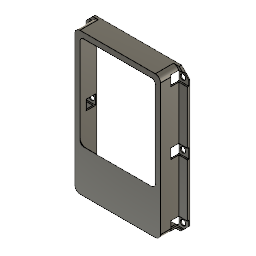
2004699B-exact (Autodesk Fusion 360 design; units mm, degrees)
Autodesk Fusion 360 part; units mm, degrees
sketch "Front" plane through (0, 0, 0) normal (0, 1, 0) x (1, 0, 0) in component "2004699B"
  line L0 (-34.4613, 0.7342) -> (100.7673, 0.7342) construction
  line L1 (-34.854, -115.3184) -> (120.0108, -115.3184) construction
  line L2 (39.1093, -14.9122) -> (120.6654, -14.9122) construction
  line L3 (3.575, 24.5274) -> (3.575, -141.9882) construction
  line L4 (78.251, 23.8729) -> (78.251, -119.9956) construction
  line L5 (-16.7886, -108.2138) -> (88.0691, -108.2138) construction
  line L6 (-18.2286, -5.0898) -> (85.3201, -5.0898) construction
  line L7 (-8.6723, -56.6518) -> (96.0546, -56.6518) construction
  line L8 (-24.3813, -113.9722) -> (90.4255, -113.9722) construction
  line L9 (-27.0881, -0.4088) -> (83.5136, -0.4088) construction
  line L10 (10.2552, -130.527) -> (10.2552, 10.1996) construction
  line L11 (71.52, -130.1852) -> (71.52, 12.6775) construction
  line L12 (5.7848, -130.0998) -> (5.7848, 6.3546) construction
  line L13 (83.0008, -137.1267) -> (83.0008, 10.6162) construction
  line L14 (-1.2002, -137.339) -> (-1.2002, 17.644) construction
  line L15 (110.5413, -110.6956) -> (5.7848, -110.6956) construction
  line L16 (110.1974, -34.3178) -> (-2.9547, -34.3178) construction
  line L17 (102.8889, -60.7158) -> (-8.8875, -60.7158) construction
  line L18 (102.459, -52.5878) -> (-11.4669, -52.5878) construction
  line L19 (40.913, -17.1802) -> (40.913, 17.1835) construction
  line L20 (69.6478, 8.6501) -> (89.4046, -11.1067) construction
  line L21 (-5.4342, -8.9542) -> (10.2552, 6.7154) construction
  line L22 (-6.1303, -103.6453) -> (12.6902, -122.4658) construction
  line L23 (73.7302, -117.8806) -> (90.3753, -101.2137) construction
  line L24 (-2.868, -104.1498) -> (87.443, -104.1498) construction
  line L25 (-3.4391, -112.2778) -> (87.0011, -112.2778) construction
  line L26 (-3.1536, -9.1538) -> (86.0732, -9.1538) construction
  line L27 (-3.3677, -1.0258) -> (85.288, -1.0258) construction
  line L28 (10.2552, -110.6956) -> (71.52, -110.6956)
  line L29 (71.52, -110.6956) -> (71.52, -34.3178)
  line L30 (71.52, -34.3178) -> (10.2552, -34.3178)
  line L31 (10.2552, -34.3178) -> (10.2552, -110.6956)
  line L32 (-1.2002, -115.3184) -> (83.0008, -115.3184)
  line L33 (83.0008, -115.3184) -> (83.0008, 0.7342)
  line L34 (83.0008, 0.7342) -> (-1.2002, 0.7342)
  line L35 (-1.2002, 0.7342) -> (-1.2002, -115.3184)
  line L36 (76.0158, -119.9569) -> (76.0158, 9.6762) construction
  line L37 (5.7848, -115.3184) -> (76.0222, -115.3184) construction
  line L38 (76.0222, -115.3184) -> (76.0222, 0.7342) construction
  line L39 (76.0222, 0.7342) -> (5.7848, 0.7342) construction
  line L40 (5.7848, 0.7342) -> (5.7848, -115.3184) construction
  line L41 (76.0222, 0.7342) -> (5.7848, 0.7342)
  line L42 (5.7848, 0.7342) -> (5.7848, -115.3184)
  line L43 (5.7848, -115.3184) -> (76.0222, -115.3184)
  line L44 (76.0222, -115.3184) -> (76.0222, 0.7342)
  line L45 (-1.2002, -108.5588) -> (5.5429, -115.3184)
  line L46 (76.2891, -115.3184) -> (83.0008, -108.585)
  line L47 (77.5637, 0.7342) -> (83.0008, -4.7029)
  line L48 (4.2664, 0.7342) -> (-1.2002, -4.7255)
  point P0 (3.575, -108.2138)
  point P1 (78.251, -108.2138)
  point P2 (78.251, -56.6518)
  point P3 (78.251, -5.0898)
  point P4 (3.575, -5.0898)
  point P5 (3.575, -56.6518)
  dimension "d1" = 1.143
  dimension "d2" = 116.0526
  dimension "d3" = 113.5634
  dimension "d4" = 103.124
  dimension "d5" = 51.562
  dimension "d6" = 74.676
  dimension "d7" = 2.2098
  dimension "d8" = 4.4704
  dimension "d9" = 61.2648
  dimension "d10" = 84.201
  dimension "d11" = 6.985
  dimension "d12" = 76.3778
  dimension "d13" = 4.6228
  dimension "d14" = 100.4062
  dimension "d15" = 37.338
  dimension "d16" = 8.128
  dimension "d17" = 4.064
  dimension "d18" = 3.6322
  dimension "d19" = 3.6322
  dimension "d20" = 3.6322
  dimension "d21" = 3.6322
  dimension "d22" = 4.064
  dimension "d23" = 8.128
  dimension "d25" = 4.064
  dimension "d26" = 8.128
  dimension "d27" = 70.231
  constraint horizontal L0
  constraint horizontal L1
  constraint horizontal L2
  constraint perpendicular L1 L3
  constraint perpendicular L1 L4
  constraint perpendicular L4 L5
  constraint perpendicular L4 L6
  constraint perpendicular L4 L7
  constraint parallel L1 L8
  constraint perpendicular L4 L9
  constraint perpendicular L0 L10
  constraint perpendicular L1 L11
  constraint perpendicular L0 L12
  constraint perpendicular L5 L13
  constraint perpendicular L6 L14
  constraint coincident L12 L15.end
  constraint perpendicular L12 L15
  constraint perpendicular L14 L16
  constraint perpendicular L14 L17
  constraint perpendicular L14 L18
  constraint perpendicular L9 L19
  constraint coincident L10 L21.end
  constraint coincident L5 P0
  constraint coincident L3 P0
  constraint coincident L4 P1
  constraint coincident L5 P1
  constraint coincident L7 P2
  constraint coincident L4 P2
  constraint coincident L6 P3
  constraint coincident L4 P3
  constraint coincident L6 P4
  constraint coincident L3 P4
  constraint coincident L7 P5
  constraint coincident L3 P5
  constraint coincident L23 L24.end
  constraint perpendicular L13 L24
  constraint perpendicular L13 L25
  constraint perpendicular L13 L26
  constraint perpendicular L13 L27
  constraint horizontal L28
  constraint vertical L29
  constraint horizontal L30
  constraint vertical L31
  constraint coincident L16 L29.end
  constraint coincident L11 L29.end
  constraint coincident L10 L28.start
  constraint coincident L15 L28.start
  constraint horizontal L32
  constraint vertical L33
  constraint horizontal L34
  constraint vertical L35
  constraint coincident L0 L33.end
  constraint coincident L13 L33.end
  constraint coincident L1 L32.start
  constraint coincident L14 L32.start
  constraint perpendicular L0 L36
  constraint horizontal L37
  constraint vertical L38
  constraint horizontal L39
  constraint vertical L40
  constraint coincident L0 L38.end
  constraint coincident L12 L37.start
  constraint coincident L32 L37.start
  constraint horizontal L41
  constraint vertical L42
  constraint horizontal L43
  constraint vertical L44
  constraint coincident L14 L45.start
  constraint coincident L1 L45.end
  constraint coincident L22 L45.end
  constraint coincident L23 L46.start
  constraint coincident L32 L46.start
  constraint coincident L13 L46.end
  constraint coincident L20 L47.start
  constraint coincident L34 L47.start
  constraint coincident L13 L47.end
  constraint coincident L20 L47.end
  constraint coincident L34 L48.start
  constraint coincident L21 L48.start
  constraint coincident L21 L48.end
  constraint coincident L35 L48.end
  measures "d1" distance of L0 L9
  measures "d2" distance of L0 L1
  measures "d3" distance of L8 L9
  measures "d4" distance of L5 L6
  measures "d5" distance of L6 L7
  measures "d6" distance of L3 L4
  measures "d7" distance of L3 L12
  measures "d8" distance of L10 L12
  measures "d9" distance of L10 L11
  measures "d10" distance of L13 L14
  measures "d11" distance of L12 L14
  measures "d12" distance of L15 L16
  measures "d13" distance of L1 L15
  measures "d14" distance of L1 L2
  measures "d15" distance of L3 L19
  measures "d16" distance of L17 L18
  measures "d17" distance of L7 L18
  measures "d18" distance of L20 P3
  measures "d19" distance of L21 P4
  measures "d20" distance of L22 P0
  measures "d21" distance of L23 P1
  measures "d22" distance of L5 L25
  measures "d23" distance of L24 L25
  measures "d25" distance of L6 L27
  measures "d26" distance of L26 L27
  measures "d27" distance of L12 L36
extrude "Extrude1" add sketch "Front" against normal blind 17.0434 contours L32 L34 L41 L42 L43 L44 in component "2004699B"
extrude "Extrude2" add sketch "Front" against normal blind 2.0828 contours L32 L34 L35 L42 L45 L48 | L32 L33 L34 L44 L46 L47 in component "2004699B"
fillet "Fillet1" radius 4.318 4 edges at (5.7848, -9.5631, -0.7342) (76.0222, -9.5631, -0.7342) (76.0222, -9.5631, 115.3184) (5.7848, -9.5631, 115.3184) in component "2004699B"
fillet "Fillet2" radius 2.8194 4 edges at (71.52, -8.5217, 110.6956) (10.2552, -8.5217, 110.6956) (71.52, -8.5217, 34.3178) (10.2552, -8.5217, 34.3178) in component "2004699B"
hole "Hole1" at (78.251, 0, 108.2138) at (78.251, 0, 56.6518) at (78.251, 0, 5.0898) at (3.575, 0, 5.0898) at (3.575, 0, 56.6518) at (3.575, 0, 108.2138) direction (0, -1, 0) diameter 4.3434 end through all in component "2004699B"
sketch "Sketch3" plane through (0, 0, 0) normal (0, 1, 0) x (1, 0, 0) in component "2004699B"
  line L0 (88.5571, -114.1754) -> (-29.017, -114.1754) construction
  line L1 (6.9278, -119.135) -> (6.9278, -3.6092) construction
  line L2 (74.8728, -110.975) -> (74.8728, 6.1599) construction
  line L3 (95.5329, -0.4088) -> (-26.782, -0.4088) construction
  line L4 (-34.4613, 0.7342) -> (100.7673, 0.7342) construction
  line L5 (5.7848, -130.0998) -> (5.7848, 6.3546) construction
  line L6 (-34.854, -115.3184) -> (120.0108, -115.3184) construction
  line L7 (76.0158, -119.9569) -> (76.0158, 9.6762) construction
  line L8 (71.6724, -114.1754) -> (10.1282, -114.1754)
  line L9 (6.9278, -110.975) -> (6.9278, -0.4088)
  line L10 (10.1282, -0.4088) -> (71.6724, -0.4088)
  line L11 (74.8728, -3.6092) -> (74.8728, -114.1754)
  arc A0 (74.8728, -3.6092) -> (71.6724, -0.4088) centre (71.6724, -3.6092) ccw
  arc A1 (10.1282, -0.4088) -> (6.9278, -3.6092) centre (10.1282, -3.6092) ccw
  arc A2 (71.6724, -114.1754) -> (74.8728, -110.975) centre (71.6724, -110.975) ccw
  arc A3 (6.9278, -110.975) -> (10.1282, -114.1754) centre (10.1282, -110.975) ccw
  dimension "d37" = 1.143
  dimension "d38" = 1.143
  dimension "d39" = 1.143
  dimension "d40" = 1.143
  dimension "d41" = 3.2004
  dimension "d42" = 3.2004
  dimension "d43" = 3.2004
  dimension "d44" = 3.2004
  constraint horizontal L0
  constraint perpendicular L0 L1
  constraint perpendicular L0 L2
  constraint perpendicular L2 L3
  constraint horizontal L8
  constraint vertical L9
  constraint horizontal L10
  constraint vertical L11
  constraint coincident L1 L9.end
  constraint coincident L3 L9.end
  constraint coincident L2 L11.end
  constraint coincident L0 L11.end
  constraint tangent L11 A0
  constraint tangent L10 A0
  constraint coincident L9.end L10
  constraint tangent L10 A1
  constraint tangent L1 A1
  constraint coincident L11.end L8
  constraint tangent L2 A2
  constraint tangent L8 A2
  constraint tangent L8 A3
  constraint tangent L9 A3
  measures "d37" distance of L3 L4
  measures "d38" distance of L1 L5
  measures "d39" distance of L0 L6
  measures "d40" distance of L2 L7
  measures "d41" radius of A0
  measures "d42" radius of A1
  measures "d43" radius of A2
  measures "d44" radius of A3
extrude "Extrude3" cut sketch "Sketch3" against normal blind 14.986 in component "2004699B"
chamfer "Chamfer1" distance 2.032 angle 45 8 edges at (40.8876, -14.986, 34.3178) (11.081, -14.986, 35.1436) (10.2552, -14.986, 72.5067) (11.081, -14.986, 109.8698) (40.8876, -14.986, 110.6956) (70.6942, -14.986, 109.8698) (71.52, -14.986, 72.5067) (70.6942, -14.986, 35.1436) in component "2004699B"
sketch "Sketch4" plane through (83.0008, 0, 0) normal (1, 0, 0) x (0, 1, 0) in component "2004699B"
  line L0 (0, 4.7029) -> (0, 108.585)
  line L1 (0, 108.585) -> (-2.0828, 108.585)
  line L2 (-2.0828, 108.585) -> (-2.0828, 4.7029)
  line L3 (-2.0828, 4.7029) -> (0, 4.7029)
  line L4 (-0.9906, 121.8672) -> (-0.9906, -5.2486) construction
  line L5 (0, 108.2121) -> (-3.3976, 108.2121) construction
  line L6 (0, 56.644) -> (-3.817, 56.644) construction
  line L7 (0, 0) -> (-1.1062, 0) construction
  line L8 (1.8872, 112.2761) -> (-9.9271, 112.2761) construction
  line L9 (1.8112, 104.1481) -> (-10.4595, 104.1481) construction
  line L10 (1.71, 60.708) -> (-9.8241, 60.708) construction
  line L11 (2.1656, 52.58) -> (0.9254, 52.58) construction
  line L12 (0.9254, 52.58) -> (-9.5412, 52.58) construction
  line L13 (0, 5.0822) -> (-6.1548, 5.0822) construction
  line L14 (2.1892, 9.1462) -> (-10.0058, 9.1462) construction
  line L15 (2.6197, 1.0182) -> (-10.581, 1.0182) construction
  line L16 (-8.6106, 122.6091) -> (-8.6106, -10.4565) construction
  line L17 (-8.6106, 60.708) -> (-0.9906, 60.708)
  line L18 (-0.9906, 60.708) -> (-0.9906, 52.58)
  line L19 (-0.9906, 52.58) -> (-8.6106, 52.58)
  line L20 (-8.6106, 52.58) -> (-8.6106, 60.708)
  line L21 (-8.6106, 9.1462) -> (-0.9906, 9.1462)
  line L22 (-0.9906, 9.1462) -> (-0.9906, 1.0182)
  line L23 (-0.9906, 1.0182) -> (-8.6106, 1.0182)
  line L24 (-8.6106, 1.0182) -> (-8.6106, 9.1462)
  line L25 (-8.6106, 112.2761) -> (-0.9906, 112.2761)
  line L26 (-0.9906, 112.2761) -> (-0.9906, 104.1481)
  line L27 (-0.9906, 104.1481) -> (-8.6106, 104.1481)
  line L28 (-8.6106, 104.1481) -> (-8.6106, 112.2761)
  point P0 (0, 119.9956)
  dimension "d48" = 0.9906
  dimension "d49" = 4.064
  dimension "d50" = 8.128
  dimension "d51" = 4.064
  dimension "d52" = 8.128
  dimension "d54" = 4.064
  dimension "d55" = 8.128
  dimension "d56" = 7.62
  constraint parallel L2 L4
  constraint coincident L0 L5.start
  constraint perpendicular L2 L5
  constraint midpoint L0 L6.start
  constraint perpendicular L0 L6
  constraint coincident L7.start origin
  constraint perpendicular L4 L7
  constraint perpendicular L4 L8
  constraint perpendicular L2 L9
  constraint perpendicular L0 L10
  constraint perpendicular L4 L11
  constraint perpendicular L4 L12
  constraint coincident L0 L13.start
  constraint perpendicular L0 L13
  constraint perpendicular L0 L14
  constraint perpendicular L0 L15
  constraint perpendicular L12 L16
  constraint horizontal L17
  constraint vertical L18
  constraint horizontal L19
  constraint vertical L20
  constraint coincident L4 L18.end
  constraint coincident L12 L18.end
  constraint coincident L16 L17.start
  constraint coincident L10 L17.start
  constraint horizontal L21
  constraint vertical L22
  constraint horizontal L23
  constraint vertical L24
  constraint coincident L4 L22.end
  constraint coincident L15 L22.end
  constraint coincident L16 L21.start
  constraint coincident L14 L21.start
  constraint horizontal L25
  constraint vertical L26
  constraint horizontal L27
  constraint vertical L28
  constraint coincident L4 L26.end
  constraint coincident L9 L26.end
  constraint coincident L16 L25.start
  constraint coincident L8 L25.start
  measures "d48" distance of L4 P0
  measures "d49" distance of L13 L14
  measures "d50" distance of L14 L15
  measures "d51" distance of L6 L10
  measures "d52" distance of L10 L12
  measures "d54" distance of L5 L9
  measures "d55" distance of L8 L9
  measures "d56" distance of L4 L16
extrude "Extrude4" cut sketch "Sketch4" against normal through all contours L2 L3 L21 L22 L23 L24 | L2 L3 L21 L22 | L1 L2 L26 L27 | L1 L2 L25 L26 L27 L28 | L2 L17 L19 L20 | L2 L17 L18 L19 in component "2004699B"
component "2004699B" placed x (1, 0, 0) y (0, 1, 0) z (0, 0, 1) at (0, 0, 0)
equation "d41 = 0.171 in - 0.045 in"
equation "d42 = 0.171 in - 0.045 in"
equation "d43 = 0.171 in - 0.045 in"
equation "d44 = 0.171 in - 0.045 in"
